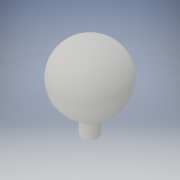
# Autodesk Inventor part: Ball
Saved by Autodesk Inventor 2017.2 (Build 212233000, 233)
## iProperties
Created: 2018-01-21
Part Number: Ball
Material: Generic
Document SubType Name: Modeling
Designer: Vatsal Varma
Density: 1 g/cm^3
Appearance: Default
Author: Vatsal Varma
Autodesk Inventor part; units mm, degrees
ref_plane "YZ Plane" through (0, 0, 0) normal (1, 0, 0) x (0, 1, 0)
ref_plane "XZ Plane" through (0, 0, 0) normal (0, 1, 0) x (-1, 0, 0)
ref_plane "XY Plane" through (0, 0, 0) normal (0, 0, 1) x (1, 0, 0)
sketch "Sketch1" plane through (0, 0, 0) normal (0, 0, 1) x (1, 0, 0)
  arc A0 (1.8824, -2.9507) -> (0, 3.5) centre (0, 0) ccw
  line L0 (1, -4.5602) -> (1, -5.7664)
  line L1 (1, -5.7664) -> (0, -5.7664)
  arc A1 (1.8824, -2.9507) -> (1, -4.5602) centre (2.9092, -4.5602) ccw
  line L2 (0, 3.5) -> (0, -5.7664)
  dimension "d0" = 7
  dimension "d1" = 1
  constraints: 6 end point, 4 point on circle, 2 centre point, 2 tangent, 1 coincident
  measures "d0" diameter of A0
  measures "d1" distance from line of L0 point (0, 0)
revolve "Revolution1" add sketch "Sketch1" angle 360 about axis through (0, 3.5, 0) along (0, -1, 0)
body "Solid1"
